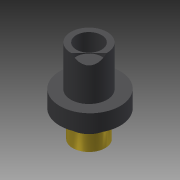
# Autodesk Inventor part: SmallConnector
Saved by Autodesk Inventor 2014 (Build 180170000, 170)
## iProperties
Created: 2015-01-07
Part Number: SmallConnector
Material: Generic
Document SubType Name: Modeling
Designer: Owner
Density: 1 g/cm^3
Appearance: Gray
Author: Owner
Autodesk Inventor part; units mm, degrees
ref_plane "YZ Plane" through (0, 0, 0) normal (1, 0, 0) x (0, 1, 0)
ref_plane "XZ Plane" through (0, 0, 0) normal (0, 1, 0) x (-1, 0, 0)
ref_plane "XY Plane" through (0, 0, 0) normal (0, 0, 1) x (1, 0, 0)
sketch "Sketch1" plane through (0, 0, 0) normal (0, 1, 0) x (-1, 0, 0)
  circle A0 centre (0, 0) radius 5.461
  dimension "d0" = 10.922
  constraints: 1 centre point, 1 coincident
  measures "d0" diameter of A0
extrude "Extrusion1" add sketch "Sketch1" along normal blind 20.066
sketch "Sketch2" plane through (0, 0, 0) normal (1, 0, 0) x (0, 1, 0)
  line L0 (2.7178, -0.3105) -> (7.8486, -0.3105)
  line L1 (7.8486, -0.3105) -> (7.8486, -9.4037)
  line L2 (7.8486, -9.4037) -> (2.7178, -9.4037)
  line L3 (2.7178, -9.4037) -> (2.7178, -0.3105)
  line L4 (0, 5.461) -> (0, -5.461) projected
  line L5 (20.066, -5.461) -> (20.066, 5.461) projected
  point P0 (0, 0)
  dimension "d3" = 9.0932
  dimension "d4" = 2.7178
  dimension "d12" = 12.2174
  constraints: 8 end point, 2 parallel, 1 horizontal, 1 perpendicular
  measures "d3" distance of L0.end L1.end
  measures "d4" distance between parallel lines of L4 L3
  measures "d12" distance between parallel lines of L5 L1
revolve "Revolution1" add sketch "Sketch2" angle 360 about axis through (0, 2.7178, -0.3105) along (0, 1, 0)
sketch "Sketch3" plane through (0, 0, 0) normal (0, -1, 0) x (1, 0, 0)
  circle A0 centre (0, 0) radius 5.461 projected
  circle A1 centre (0, 0) radius 4.8747
  constraints: 1 centre point, 1 coincident
extrude "Extrusion2" add sketch "Sketch3" along normal blind 5.08 contours A1
sketch "Sketch4" plane through (0, 20.066, 0) normal (0, 1, 0) x (1, 0, 0)
  circle A0 centre (0, 0) radius 5.461 projected
  circle A1 centre (0, 0) radius 3.81
  dimension "d9" = 7.62
  constraints: 1 centre point, 1 coincident
  measures "d9" diameter of A1
extrude "Extrusion3" cut sketch "Sketch4" against normal blind 5.588 contours A1
body "Solid1"
